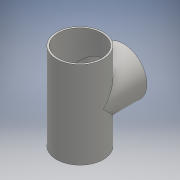
# Autodesk Inventor part: têe 10 inch ANSI B16.9
Saved by Autodesk Inventor 2016 (Build 200138000, 138)
## iProperties
Created: 2019-01-09
Part Number: têe 10 inch ANSI B16.9
Material: Generic
Document SubType Name: Modeling
Designer: Cliente
Density: 1 g/cm^3
Appearance: Default
Author: Cliente
Autodesk Inventor part; units mm, degrees
ref_plane "YZ Plane" through (0, 0, 0) normal (1, 0, 0) x (0, 1, 0)
ref_plane "XZ Plane" through (0, 0, 0) normal (0, 1, 0) x (-1, 0, 0)
ref_plane "XY Plane" through (0, 0, 0) normal (0, 0, 1) x (1, 0, 0)
sketch "Sketch1" plane through (0, 0, 0) normal (0, 0, 1) x (1, 0, 0)
  circle A0 centre (0, 0) radius 136.5
  circle A1 centre (0, 0) radius 126.98
  dimension "d0" = 273
  dimension "d1" = 9.52
  constraints: 2 centre point, 2 coincident
  measures "d0" diameter of A0
  measures "d1" radial gap between concentric circles of A0 A1
extrude "Extrusion1" add sketch "Sketch1" along normal mid plane 508
sketch "Sketch2" plane through (0, 0, 0) normal (0, 1, 0) x (-1, 0, 0)
  circle A0 centre (0, 0) radius 136.5
  circle A1 centre (0, 0) radius 126.98
  dimension "d4" = 9.52
  dimension "d5" = 273
  constraints: 2 centre point, 2 coincident
  measures "d4" radial gap between concentric circles of A0 A1
  measures "d5" diameter of A0
extrude "Extrusion2" add sketch "Sketch2" along normal blind 254
sketch "Sketch3" plane through (0, 0, 254) normal (0, 0, 1) x (1, 0, 0)
  circle A0 centre (0, 0) radius 126.98 projected
extrude "Extrusion3" cut sketch "Sketch3" against normal through all
sketch "Sketch4" plane through (0, 254, 0) normal (0, 1, 0) x (1, 0, 0)
  spline S0 degree 2 poles (-126.98, 0) (-126.98, -219.9358) (63.49, -109.9679) (253.96, 0) (63.49, 109.9679) (-126.98, 219.9358) (-126.98, 0) knots 0 0 0 0.333333 0.333333 0.666667 0.666667 1 1 1 weights 1 0.5 1 0.5 1 0.5 1 projected
  arc A0 (136.5, 0) -> (-136.5, 0) centre (0, 0) ccw projected
  constraints: 1 horizontal alignment, 1 other
extrude "Extrusion4" cut sketch "Sketch4" against normal blind 254
body "Solid1"
